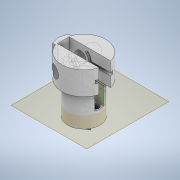
# Autodesk Inventor part: handle_base
Saved by Autodesk Inventor 2021 (Build 250183000, 183)
## iProperties
Created: 2021-03-06
Part Number: handle_base
Material: Generic
Document SubType Name: Modeling
Designer: ben
Density: 1 g/cm^3
Appearance: Default
Mass: 226.368 g
Surface Area: 425.082 cm^2
Volume: 226.368 cm^3
Author: ben
Autodesk Inventor part; units mm, degrees
ref_plane "YZ Plane" through (0, 0, 0) normal (1, 0, 0) x (0, 1, 0)
ref_plane "XZ Plane" through (0, 0, 0) normal (0, 1, 0) x (-1, 0, 0)
ref_plane "XY Plane" through (0, 0, 0) normal (0, 0, 1) x (1, 0, 0)
ref_plane "Work Plane1" through (-35, 22.5, -35) normal (0, 0, 1) x (1, 0, 0)
sketch "Sketch1" plane through (-35, 22.5, -35) normal (0, 0, 1) x (1, 0, 0)
  circle A0 centre (35, -42) radius 27.5
  circle A1 centre (35, -42) radius 6
  circle A2 centre (15, -42) radius 6
  point P0 (35, -22.5)
  dimension "d0" = 55
  dimension "d24" = 12
  dimension "d50" = 12
  constraints: 3 centre point, 1 coincident
  measures "d0" diameter of A0
  measures "d24" diameter of A1
  measures "d50" diameter of A2
ref_plane "Work Plane2" through (0, -19.5, 0) normal (0, 0, 1) x (1, 0, 0)
sketch "Sketch2" plane through (0, -19.5, 0) normal (0, 0, 1) x (1, 0, 0)
  arc A0 (-36.1421, -10) -> (-36.1421, 10) centre (0, 0) ccw
  line L0 (37.5, -10) -> (-36.1421, -10)
  line L1 (-36.1421, 10) -> (37.5, 10)
  line L2 (37.5, 10) -> (37.5, -10)
  line L3 (34.9857, -13.5) -> (39.9857, -13.5)
  line L4 (39.9857, -13.5) -> (39.9857, 13.5)
  line L5 (39.9857, 13.5) -> (34.9857, 13.5)
  line L6 (34.9857, 13.5) -> (34.9857, -13.5)
  line L7 (39.9857, -13.5) -> (43.6938, 0)
  line L8 (43.6938, 0) -> (39.9857, 13.5)
  point P0 (0, 19.5)
  point P1 (37.5, 0)
  point P2 (36.1421, 10)
  point P3 (36.1421, -10)
  point P4 (34.9857, 10)
  point P5 (34.9857, -10)
  dimension "d3" = 75
  dimension "d40" = 5
  dimension "d41" = 27
  dimension "d44" = 14
  constraints: 18 end point, 4 horizontal, 4 point on circle, 3 parallel, 1 centre point, 1 perpendicular, 1 tangent, 1 vertical, 1 other
  measures "d3" diameter of A0
  measures "d40" distance of L3.start L3.end
  measures "d41" distance of L5.end L3.start
  measures "d44" distance of L3.end L7.end
extrude "Extrusion2" add sketch "Sketch2" along normal blind 40
ref_plane "Work Plane3" through (-36.1421, -9.5, 0) normal (0, -1, 0) x (1, 0, 0)
sketch "Sketch4" plane through (-36.1421, -9.5, 0) normal (0, -1, 0) x (1, 0, 0)
  line L0 (0, 0) -> (10.5247, 0) projected
  point P0 (36.1421, 0)
  point P1 (51.9367, 20)
hole "Hole2" at (15.7946, -9.5, 20) direction (0, 1, 0) diameter 19.05 end through all both
extrude "Extrusion3" add sketch "Sketch1" along normal blind 35 and the other way blind 20
sketch "Sketch8" plane through (0, -19.5, -55) normal (0, 0, -1) x (-1, 0, 0)
  circle A0 centre (0, 0) radius 6 projected
  circle A1 centre (0, 0) radius 6 projected
  line L0 (-6, 10.3923) -> (12, 0)
  line L1 (12, 0) -> (-6, -10.3923)
  line L2 (-6, -10.3923) -> (-6, 10.3923)
  point P0 (0, 19.5)
  point P1 (-6, 0)
  constraints: 6 end point, 1 coincident, 1 horizontal alignment, 1 midpoint, 8 other
extrude "Extrusion5" add sketch "Sketch8" along normal blind 15
sketch "Sketch10" plane through (-35, 22.5, 0) normal (0, 0, 1) x (1, 0, 0)
  arc A0 (9.3826, -32) -> (9.3826, -52) centre (35, -42) ccw projected
  line L0 (7.5, -42) -> (7.5, -52)
  line L1 (7.5, -42) -> (7.5, -32)
  line L2 (-1.1421, -32) -> (69.9857, -32) projected
  line L3 (7.5, -34.5) -> (43.9, -34.5)
  line L4 (43.9, -34.5) -> (43.9, -49.5)
  line L5 (43.9, -49.5) -> (7.5, -49.5)
  line L6 (7.5, -49.5) -> (7.5, -34.5)
  point P0 (35, -22.5)
  point P1 (8.5425, -34.5)
  point P2 (8.5425, -49.5)
  point P3 (71.1421, -32)
  dimension "d45" = 36.4
  dimension "d46" = 15
  constraints: 12 end point, 2 parallel, 2 point on line, 2 vertical, 1 horizontal, 1 perpendicular, 1 point on circle, 1 tangent
  measures "d45" distance of L4.end L5.end
  measures "d46" distance of L3.end L4.end
extrude "Extrusion7" cut sketch "Sketch10" against normal blind 30.7 contours L3 L4 L5 A0
ref_plane "Work Plane4" through (-35, 22.5, 0) normal (0, 0, 1) x (1, 0, 0)
split body "Split1" result two bodies by plane through (-35, 22.5, 0) normal (0, 0, 1) first body at (28.9114, 3.5897, 20.1633)
sketch "Sketch11" plane through (0, -19.5, -55) normal (0, 0, -1) x (-1, 0, 0)
  circle A0 centre (20, 0) radius 6 projected
  circle A1 centre (0, 0) radius 6 projected
  point P0 (0, 19.5)
extrude "Extrusion8" add sketch "Sketch11" against normal blind 10 bodies 3
sketch "Sketch13" plane through (-36.1421, -29.5, 0) normal (0, 1, 0) x (1, 0, 0)
  line L0 (40, -20) -> (40, -20)
  circle A0 centre (51.9367, -20) radius 9.525 projected
  line L1 (34.9997, -20) -> (0, -20) construction
  line L2 (0, 0) -> (0, -40) projected
  line L3 (34.9997, -17.5) -> (0, -17.5)
  line L4 (0, -22.5) -> (32.6611, -22.5)
  arc A1 (0, -17.5) -> (0, -22.5) centre (0, -20) ccw
  arc A2 (37.4997, -20) -> (41.7282, -30.2085) centre (51.9367, -20) ccw
  line L5 (51.9367, -20) -> (41.7282, -30.2085) construction
  line L6 (51.9367, -20) -> (37.4997, -20) construction
  arc A3 (32.6611, -22.5) -> (38.1927, -33.744) centre (51.9367, -20) ccw
  line L7 (51.9367, -20) -> (38.1927, -33.744) construction
  line L8 (51.9367, -20) -> (32.4997, -20) construction
  arc A4 (38.1927, -33.744) -> (41.7282, -30.2085) centre (39.9604, -31.9763) ccw
  line L9 (37.4997, -20) -> (37.4997, -17.5)
  line L10 (37.4997, -17.5) -> (34.9997, -17.5)
  point P0 (36.1421, 0)
  point P1 (17.4998, -20)
  dimension "d61" = 5
  dimension "d62" = 45
  dimension "d63" = 19.437
  dimension "d64" = 45
  dimension "d65" = 40
  dimension "d66" = 22.5
  dimension "d67" = 2.5
  dimension "d68" = 2.5
  constraints: 22 end point, 9 point on circle, 4 centre point, 3 point on line, 3 tangent, 2 coincident, 2 midpoint, 1 collinear, 1 equal radius, 1 parallel, 1 perpendicular, 1 vertical
  measures "d61" diameter of A1
  measures "d62" angle of L6 L5
  measures "d63" radius of A3
  measures "d64" angle of L8 L7
  measures "d65" distance from line of L2.end L0
  measures "d66" distance from line of L2.end L3
  measures "d67" distance from line of L0.end L3
  measures "d68" distance from line of L0.start L3
extrude "Extrusion9" cut sketch "Sketch13" along normal blind 25 and the other way blind 5 contours L3 L10 L9 A2 A4 A3 L4 L2 bodies 2
